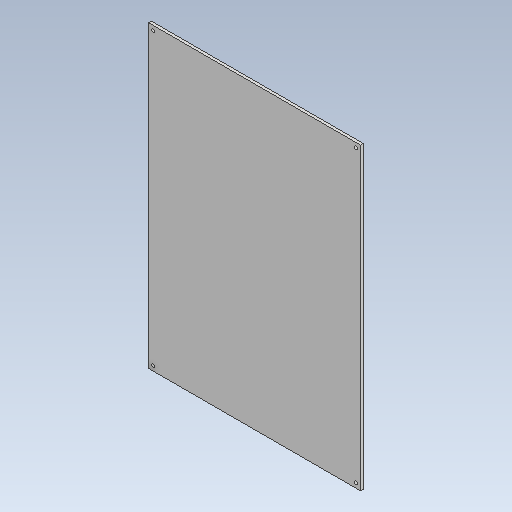
# Autodesk Inventor part: 0005-10-013 Bed
Saved by Autodesk Inventor 2020 (Build 240168000, 168)
## iProperties
Created: 2020-12-19
Part Number: 0005-10-013 Bed
Material: Generic
Document SubType Name: Modeling
Designer: Iulian Bors
Density: 1 g/cm^3
Appearance: Default
Author: Iulian Bors
Subject: 013
Autodesk Inventor part; units mm, degrees
ref_plane "YZ Plane" through (0, 0, 0) normal (1, 0, 0) x (0, 1, 0)
ref_plane "XZ Plane" through (0, 0, 0) normal (0, 1, 0) x (-1, 0, 0)
ref_plane "XY Plane" through (0, 0, 0) normal (0, 0, 1) x (1, 0, 0)
sketch "Sketch1" plane through (0, 0, 0) normal (0, 0, 1) x (1, 0, 0)
  line L0 (-115, 162.5) -> (115, 162.5)
  line L1 (115, 162.5) -> (115, -162.5)
  line L2 (115, -162.5) -> (-115, -162.5)
  line L3 (-115, -162.5) -> (-115, 162.5)
  point P0 (0, 0)
  point P1 (0, 162.5)
  point P2 (-115, 0)
  dimension "d0" = 230
  dimension "d1" = 325
  constraints: 8 end point, 2 midpoint, 2 parallel, 1 horizontal, 1 horizontal alignment, 1 perpendicular, 1 vertical alignment
  measures "d0" distance of L0.start L0.end
  measures "d1" distance of L0.end L1.end
extrude "Extrusion1" add sketch "Sketch1" along normal blind 3
sketch "Sketch2" plane through (0, 0, 3) normal (0, 0, 1) x (1, 0, 0)
  line L0 (-110, -157.5) -> (110, -157.5) construction
  line L1 (110, -157.5) -> (110, 157.5) construction
  line L2 (110, 157.5) -> (-110, 157.5) construction
  line L3 (-110, 157.5) -> (-110, -157.5) construction
  line L4 (-115, 162.5) -> (-115, -162.5) construction
  line L5 (115, 162.5) -> (-115, 162.5) construction
  point P0 (0, 0)
  point P1 (-110, 0)
  point P2 (-115, 0)
  point P3 (-115, 0)
  point P4 (0, 157.5)
  point P5 (0, 162.5)
  dimension "d4" = 5
  dimension "d5" = 5
  constraints: 8 end point, 5 midpoint, 4 coincident, 2 parallel, 1 horizontal, 1 horizontal alignment, 1 perpendicular, 1 vertical alignment
  measures "d4" distance between parallel lines of L4 L3
  measures "d5" distance between parallel lines of L5 L2
hole "Hole1" at (-110, -157.5, 3) at (-110, 157.5, 3) at (110, 157.5, 3) at (110, -157.5, 3) direction (0, 0, -1) diameter 3.5 end through all
body "Solid1"
